Autodesk Fusion 360 part; units mm, degrees
note: some values were not read from the file. Set by a fixed rule: the direction of a hole.
(part 2 of 10)
  line L984 (55.9165, 3.84) -> (55.9165, 5.94)
  line L985 (53.6861, 6.8639) -> (53.4029, 6.44)
  line L986 (53.3035, 5.94) -> (53.3035, 5.94)
  line L987 (53.3035, 3.84) -> (53.3035, 3.84)
  line L988 (55.8171, 6.44) -> (55.5339, 6.8639)
  line L989 (55.5339, 6.8639) -> (55.11, 7.1471)
  line L990 (53.4029, 6.44) -> (53.3035, 5.94)
  line L991 (53.3035, 5.94) -> (53.3035, 3.84)
  line L992 (53.4029, 3.34) -> (53.6861, 2.9161)
  line L993 (55.11, 2.6329) -> (55.5339, 2.9161)
  line L994 (55.9165, 5.94) -> (55.9165, 5.94)
  line L995 (54.61, 7.2465) -> (54.11, 7.1471)
  line L996 (55.11, 7.1471) -> (54.61, 7.2465)
  line L997 (55.5339, 2.9161) -> (55.8171, 3.34)
  line L998 (53.3035, 3.84) -> (53.4029, 3.34)
  line L999 (96.49, 12.1015) -> (96.49, 12.1015)
  line L1000 (94.39, 9.4885) -> (96.49, 9.4885)
  line L1001 (93.1829, 11.295) -> (93.0835, 10.795)
  line L1002 (93.4661, 11.7189) -> (93.1829, 11.295)
  line L1003 (94.39, 12.1015) -> (93.89, 12.0021)
  line L1004 (93.89, 9.5879) -> (94.39, 9.4885)
  line L1005 (93.4661, 9.8711) -> (93.89, 9.5879)
  line L1006 (93.0835, 10.795) -> (93.1829, 10.295)
  line L1007 (93.1829, 10.295) -> (93.4661, 9.8711)
  line L1008 (96.99, 9.5879) -> (97.4139, 9.8711)
  line L1009 (97.6971, 10.295) -> (97.7965, 10.795)
  line L1010 (96.99, 12.0021) -> (96.49, 12.1015)
  line L1011 (96.49, 12.1015) -> (94.39, 12.1015)
  line L1012 (96.49, 9.4885) -> (96.49, 9.4885)
  line L1013 (94.39, 12.1015) -> (94.39, 12.1015)
  line L1014 (97.4139, 9.8711) -> (97.6971, 10.295)
  line L1015 (97.7965, 10.795) -> (97.6971, 11.295)
  line L1016 (93.89, 12.0021) -> (93.4661, 11.7189)
  line L1017 (94.39, 9.4885) -> (94.39, 9.4885)
  line L1018 (96.49, 9.4885) -> (96.99, 9.5879)
  line L1019 (97.4139, 11.7189) -> (96.99, 12.0021)
  line L1020 (97.6971, 11.295) -> (97.4139, 11.7189)
  line L1021 (67.81, 2.6329) -> (68.2339, 2.9161)
  line L1022 (67.31, 2.5335) -> (67.81, 2.6329)
  line L1023 (66.1029, 3.34) -> (66.3861, 2.9161)
  line L1024 (68.2339, 2.9161) -> (68.5171, 3.34)
  line L1025 (66.3861, 6.8639) -> (66.1029, 6.44)
  line L1026 (68.6165, 3.84) -> (68.6165, 3.84)
  line L1027 (66.3861, 2.9161) -> (66.81, 2.6329)
  line L1028 (67.31, 7.2465) -> (66.81, 7.1471)
  line L1029 (68.5171, 3.34) -> (68.6165, 3.84)
  line L1030 (66.0035, 5.94) -> (66.0035, 3.84)
  line L1031 (66.81, 2.6329) -> (67.31, 2.5335)
  line L1032 (68.6165, 5.94) -> (68.6165, 5.94)
  line L1033 (66.81, 7.1471) -> (66.3861, 6.8639)
  line L1034 (66.0035, 3.84) -> (66.0035, 3.84)
  line L1035 (67.81, 7.1471) -> (67.31, 7.2465)
  line L1036 (68.6165, 3.84) -> (68.6165, 5.94)
  line L1037 (66.1029, 6.44) -> (66.0035, 5.94)
  line L1038 (66.0035, 3.84) -> (66.1029, 3.34)
  line L1039 (66.0035, 5.94) -> (66.0035, 5.94)
  line L1040 (68.5171, 6.44) -> (68.2339, 6.8639)
  line L1041 (68.6165, 5.94) -> (68.5171, 6.44)
  line L1042 (68.2339, 6.8639) -> (67.81, 7.1471)
  line L1043 (41.9076, 68.8233) -> (41.9076, 68.8233)
  line L1044 (43.1725, 69.5114) -> (43.1997, 69.6484)
  line L1045 (43.1997, 70.1154) -> (43.1997, 70.1154)
  line L1046 (41.6544, 68.9282) -> (41.7706, 68.8506)
  line L1047 (43.1997, 69.6484) -> (43.1997, 70.1154)
  line L1048 (42.6278, 68.9282) -> (42.6278, 68.9282)
  line L1049 (41.7706, 68.8506) -> (41.9076, 68.8233)
  line L1050 (42.6278, 70.8356) -> (42.5117, 70.9132)
  line L1051 (43.0948, 70.3686) -> (43.0948, 70.3686)
  line L1052 (41.1874, 69.3952) -> (41.6544, 68.9282)
  line L1053 (41.1098, 70.2525) -> (41.0825, 70.1154)
  line L1054 (41.9076, 68.8233) -> (42.3746, 68.8233)
  line L1055 (43.1725, 70.2525) -> (43.0948, 70.3686)
  line L1056 (43.1997, 69.6484) -> (43.1997, 69.6484)
  line L1057 (42.3746, 68.8233) -> (42.5117, 68.8506)
  line L1058 (42.3746, 68.8233) -> (42.3746, 68.8233)
  line L1059 (43.1997, 70.1154) -> (43.1725, 70.2525)
  line L1060 (41.6544, 68.9282) -> (41.6544, 68.9282)
  line L1061 (41.0825, 69.6484) -> (41.1098, 69.5114)
  line L1062 (42.5117, 70.9132) -> (42.3746, 70.9405)
  line L1063 (43.0948, 70.3686) -> (42.6278, 70.8356)
  line L1064 (41.0825, 70.1154) -> (41.0825, 69.6484)
  line L1065 (41.6544, 70.8356) -> (41.1874, 70.3686)
  line L1066 (41.1874, 69.3952) -> (41.1874, 69.3952)
  line L1067 (41.6544, 70.8356) -> (41.6544, 70.8356)
  line L1068 (41.7706, 70.9132) -> (41.6544, 70.8356)
  line L1069 (42.3746, 70.9405) -> (42.3746, 70.9405)
  line L1070 (41.0825, 70.1154) -> (41.0825, 70.1154)
  line L1071 (41.1874, 70.3686) -> (41.1874, 70.3686)
  line L1072 (42.5117, 68.8506) -> (42.6278, 68.9282)
  line L1073 (41.1098, 69.5114) -> (41.1874, 69.3952)
  line L1074 (41.1874, 70.3686) -> (41.1098, 70.2525)
  line L1075 (41.0825, 69.6484) -> (41.0825, 69.6484)
  line L1076 (42.3746, 70.9405) -> (41.9076, 70.9405)
  line L1077 (41.9076, 70.9405) -> (41.9076, 70.9405)
  line L1078 (42.6278, 70.8356) -> (42.6278, 70.8356)
  line L1079 (43.0948, 69.3952) -> (43.1725, 69.5114)
  line L1080 (42.6278, 68.9282) -> (43.0948, 69.3952)
  line L1081 (41.9076, 70.9405) -> (41.7706, 70.9132)
  line L1082 (43.0948, 69.3952) -> (43.0948, 69.3952)
  line L1083 (35.9106, 76.5794) -> (35.9882, 76.6956)
  line L1084 (33.9256, 76.6956) -> (34.0032, 76.5794)
  line L1085 (35.4436, 78.0198) -> (35.4436, 78.0198)
  line L1086 (35.3275, 76.0348) -> (35.4436, 76.1124)
  line L1087 (34.4702, 76.1124) -> (34.4702, 76.1124)
  line L1088 (34.4702, 76.1124) -> (34.5864, 76.0348)
  line L1089 (35.1904, 78.1247) -> (35.1904, 78.1247)
  line L1090 (34.0032, 76.5794) -> (34.4702, 76.1124)
  line L1091 (35.9882, 76.6956) -> (36.0155, 76.8326)
  line L1092 (35.4436, 78.0198) -> (35.3275, 78.0975)
  line L1093 (35.4436, 76.1124) -> (35.9106, 76.5794)
  line L1094 (33.9256, 77.4367) -> (33.8983, 77.2996)
  line L1095 (34.7234, 76.0075) -> (34.7234, 76.0075)
  line L1096 (35.9106, 76.5794) -> (35.9106, 76.5794)
  line L1097 (35.9106, 77.5528) -> (35.9106, 77.5528)
  line L1098 (36.0155, 76.8326) -> (36.0155, 76.8326)
  line L1099 (34.0032, 77.5528) -> (33.9256, 77.4367)
  line L1100 (34.4702, 78.0198) -> (34.4702, 78.0198)
  line L1101 (36.0155, 77.2996) -> (35.9882, 77.4367)
  line L1102 (34.7234, 78.1247) -> (34.7234, 78.1247)
  line L1103 (35.3275, 78.0975) -> (35.1904, 78.1247)
  line L1104 (33.8983, 76.8326) -> (33.8983, 76.8326)
  line L1105 (35.1904, 78.1247) -> (34.7234, 78.1247)
  line L1106 (34.7234, 76.0075) -> (35.1904, 76.0075)
  line L1107 (35.9882, 77.4367) -> (35.9106, 77.5528)
  line L1108 (34.4702, 78.0198) -> (34.0032, 77.5528)
  line L1109 (36.0155, 77.2996) -> (36.0155, 77.2996)
  line L1110 (33.8983, 77.2996) -> (33.8983, 77.2996)
  line L1111 (33.8983, 77.2996) -> (33.8983, 76.8326)
  line L1112 (35.9106, 77.5528) -> (35.4436, 78.0198)
  line L1113 (35.1904, 76.0075) -> (35.1904, 76.0075)
  line L1114 (35.1904, 76.0075) -> (35.3275, 76.0348)
  line L1115 (33.8983, 76.8326) -> (33.9256, 76.6956)
  line L1116 (36.0155, 76.8326) -> (36.0155, 77.2996)
  line L1117 (34.7234, 78.1247) -> (34.5864, 78.0975)
  line L1118 (34.5864, 76.0348) -> (34.7234, 76.0075)
  line L1119 (34.0032, 76.5794) -> (34.0032, 76.5794)
  line L1120 (34.0032, 77.5528) -> (34.0032, 77.5528)
  line L1121 (34.5864, 78.0975) -> (34.4702, 78.0198)
  line L1122 (92.0234, 77.1136) -> (91.9073, 77.1913)
  line L1123 (90.4215, 76.5302) -> (90.4215, 75.8698)
  line L1124 (90.8566, 75.2864) -> (90.8566, 75.2864)
  line L1125 (90.9727, 77.1913) -> (90.8566, 77.1136)
  line L1126 (90.8566, 75.2864) -> (90.9727, 75.2087)
  line L1127 (90.8566, 77.1136) -> (90.8566, 77.1136)
  line L1128 (90.9727, 75.2087) -> (91.1098, 75.1815)
  line L1129 (90.5264, 75.6166) -> (90.5264, 75.6166)
  line L1130 (91.7702, 77.2185) -> (91.7702, 77.2185)
  line L1131 (92.3536, 75.6166) -> (92.3536, 75.6166)
  line L1132 (90.4487, 76.6673) -> (90.4215, 76.5302)
  line L1133 (91.1098, 75.1815) -> (91.1098, 75.1815)
  line L1134 (91.7702, 75.1815) -> (91.9073, 75.2087)
  line L1135 (90.4215, 75.8698) -> (90.4215, 75.8698)
  line L1136 (91.1098, 77.2185) -> (90.9727, 77.1913)
  line L1137 (90.4487, 75.7327) -> (90.5264, 75.6166)
  line L1138 (90.5264, 76.7834) -> (90.5264, 76.7834)
  line L1139 (91.1098, 75.1815) -> (91.7702, 75.1815)
  line L1140 (92.4585, 75.8698) -> (92.4585, 76.5302)
  line L1141 (91.7702, 75.1815) -> (91.7702, 75.1815)
  line L1142 (90.5264, 75.6166) -> (90.8566, 75.2864)
  line L1143 (92.4313, 75.7327) -> (92.4585, 75.8698)
  line L1144 (90.4215, 76.5302) -> (90.4215, 76.5302)
  line L1145 (92.0234, 75.2864) -> (92.0234, 75.2864)
  line L1146 (92.3536, 75.6166) -> (92.4313, 75.7327)
  line L1147 (91.9073, 75.2087) -> (92.0234, 75.2864)
  line L1148 (92.0234, 75.2864) -> (92.3536, 75.6166)
  line L1149 (90.8566, 77.1136) -> (90.5264, 76.7834)
  line L1150 (92.4585, 76.5302) -> (92.4313, 76.6673)
  line L1151 (91.7702, 77.2185) -> (91.1098, 77.2185)
  line L1152 (92.3536, 76.7834) -> (92.0234, 77.1136)
  line L1153 (91.9073, 77.1913) -> (91.7702, 77.2185)
  line L1154 (90.5264, 76.7834) -> (90.4487, 76.6673)
  line L1155 (91.1098, 77.2185) -> (91.1098, 77.2185)
  line L1156 (92.4585, 75.8698) -> (92.4585, 75.8698)
  line L1157 (90.4215, 75.8698) -> (90.4487, 75.7327)
  line L1158 (92.4313, 76.6673) -> (92.3536, 76.7834)
  line L1159 (92.4585, 76.5302) -> (92.4585, 76.5302)
  line L1160 (92.3536, 76.7834) -> (92.3536, 76.7834)
  line L1161 (92.0234, 77.1136) -> (92.0234, 77.1136)
  line L1162 (77.7215, 75.8698) -> (77.7215, 75.8698)
  line L1163 (78.1566, 75.2864) -> (78.2727, 75.2087)
  line L1164 (77.7487, 75.7327) -> (77.8264, 75.6166)
  line L1165 (78.1566, 77.1136) -> (77.8264, 76.7834)
  line L1166 (77.8264, 75.6166) -> (78.1566, 75.2864)
  line L1167 (79.3234, 75.2864) -> (79.6536, 75.6166)
  line L1168 (77.8264, 76.7834) -> (77.7487, 76.6673)
  line L1169 (77.7215, 76.5302) -> (77.7215, 75.8698)
  line L1170 (79.0702, 77.2185) -> (78.4098, 77.2185)
  line L1171 (79.6536, 75.6166) -> (79.6536, 75.6166)
  line L1172 (78.1566, 77.1136) -> (78.1566, 77.1136)
  line L1173 (79.3234, 77.1136) -> (79.3234, 77.1136)
  line L1174 (78.1566, 75.2864) -> (78.1566, 75.2864)
  line L1175 (79.7313, 75.7327) -> (79.7585, 75.8698)
  line L1176 (78.4098, 75.1815) -> (78.4098, 75.1815)
  line L1177 (78.2727, 77.1913) -> (78.1566, 77.1136)
  line L1178 (77.8264, 75.6166) -> (77.8264, 75.6166)
  line L1179 (79.6536, 76.7834) -> (79.6536, 76.7834)
  line L1180 (79.6536, 75.6166) -> (79.7313, 75.7327)
  line L1181 (78.4098, 75.1815) -> (79.0702, 75.1815)
  line L1182 (78.2727, 75.2087) -> (78.4098, 75.1815)
  line L1183 (79.7585, 76.5302) -> (79.7313, 76.6673)
  line L1184 (79.7585, 76.5302) -> (79.7585, 76.5302)
  line L1185 (79.0702, 77.2185) -> (79.0702, 77.2185)
  line L1186 (79.3234, 77.1136) -> (79.2073, 77.1913)
  line L1187 (77.7215, 76.5302) -> (77.7215, 76.5302)
  line L1188 (79.7585, 75.8698) -> (79.7585, 75.8698)
  line L1189 (77.8264, 76.7834) -> (77.8264, 76.7834)
  line L1190 (79.3234, 75.2864) -> (79.3234, 75.2864)
  line L1191 (79.0702, 75.1815) -> (79.0702, 75.1815)
  line L1192 (77.7215, 75.8698) -> (77.7487, 75.7327)
  line L1193 (79.7585, 75.8698) -> (79.7585, 76.5302)
  line L1194 (77.7487, 76.6673) -> (77.7215, 76.5302)
  line L1195 (79.2073, 77.1913) -> (79.0702, 77.2185)
  line L1196 (78.4098, 77.2185) -> (78.2727, 77.1913)
  line L1197 (78.4098, 77.2185) -> (78.4098, 77.2185)
  line L1198 (79.7313, 76.6673) -> (79.6536, 76.7834)
  line L1199 (79.2073, 75.2087) -> (79.3234, 75.2864)
  line L1200 (79.0702, 75.1815) -> (79.2073, 75.2087)
  line L1201 (79.6536, 76.7834) -> (79.3234, 77.1136)
  line L1202 (81.8634, 75.2864) -> (81.8634, 75.2864)
  line L1203 (80.2887, 76.6673) -> (80.2615, 76.5302)
  line L1204 (82.1936, 75.6166) -> (82.1936, 75.6166)
  line L1205 (81.7473, 75.2087) -> (81.8634, 75.2864)
  line L1206 (82.2713, 76.6673) -> (82.1936, 76.7834)
  line L1207 (81.6102, 75.1815) -> (81.7473, 75.2087)
  line L1208 (80.9498, 77.2185) -> (80.9498, 77.2185)
  line L1209 (80.2615, 76.5302) -> (80.2615, 76.5302)
  line L1210 (80.8127, 75.2087) -> (80.9498, 75.1815)
  line L1211 (80.6966, 75.2864) -> (80.8127, 75.2087)
  line L1212 (80.9498, 75.1815) -> (80.9498, 75.1815)
  line L1213 (81.6102, 77.2185) -> (81.6102, 77.2185)
  line L1214 (80.6966, 75.2864) -> (80.6966, 75.2864)
  line L1215 (81.6102, 77.2185) -> (80.9498, 77.2185)
  line L1216 (81.8634, 75.2864) -> (82.1936, 75.6166)
  line L1217 (82.2985, 75.8698) -> (82.2985, 76.5302)
  line L1218 (80.2615, 76.5302) -> (80.2615, 75.8698)
  line L1219 (80.8127, 77.1913) -> (80.6966, 77.1136)
  line L1220 (81.8634, 77.1136) -> (81.8634, 77.1136)
  line L1221 (82.2985, 76.5302) -> (82.2713, 76.6673)
  line L1222 (81.8634, 77.1136) -> (81.7473, 77.1913)
  line L1223 (80.3664, 75.6166) -> (80.6966, 75.2864)
  line L1224 (81.6102, 75.1815) -> (81.6102, 75.1815)
  line L1225 (80.3664, 76.7834) -> (80.2887, 76.6673)
  line L1226 (80.9498, 75.1815) -> (81.6102, 75.1815)
  line L1227 (80.3664, 75.6166) -> (80.3664, 75.6166)
  line L1228 (80.6966, 77.1136) -> (80.6966, 77.1136)
  line L1229 (82.2985, 76.5302) -> (82.2985, 76.5302)
  line L1230 (80.2887, 75.7327) -> (80.3664, 75.6166)
  line L1231 (80.2615, 75.8698) -> (80.2887, 75.7327)
  line L1232 (80.9498, 77.2185) -> (80.8127, 77.1913)
  line L1233 (81.7473, 77.1913) -> (81.6102, 77.2185)
  line L1234 (82.1936, 76.7834) -> (81.8634, 77.1136)
  line L1235 (80.6966, 77.1136) -> (80.3664, 76.7834)
  line L1236 (80.2615, 75.8698) -> (80.2615, 75.8698)
  line L1237 (82.1936, 76.7834) -> (82.1936, 76.7834)
  line L1238 (82.2985, 75.8698) -> (82.2985, 75.8698)
  line L1239 (82.1936, 75.6166) -> (82.2713, 75.7327)
  line L1240 (80.3664, 76.7834) -> (80.3664, 76.7834)
  line L1241 (82.2713, 75.7327) -> (82.2985, 75.8698)
  line L1242 (89.7027, 15.5187) -> (89.8398, 15.4915)
  line L1243 (89.1515, 16.8402) -> (89.1515, 16.1798)
  line L1244 (89.5866, 17.4236) -> (89.2564, 17.0934)
  line L1245 (89.5866, 17.4236) -> (89.5866, 17.4236)
  line L1246 (89.7027, 17.5013) -> (89.5866, 17.4236)
  line L1247 (90.6373, 17.5013) -> (90.5002, 17.5285)
  line L1248 (89.2564, 15.9266) -> (89.2564, 15.9266)
  line L1249 (89.1787, 16.9773) -> (89.1515, 16.8402)
  line L1250 (89.8398, 17.5285) -> (89.7027, 17.5013)
  line L1251 (89.2564, 17.0934) -> (89.1787, 16.9773)
  line L1252 (89.2564, 17.0934) -> (89.2564, 17.0934)
  line L1253 (89.1515, 16.1798) -> (89.1787, 16.0427)
  line L1254 (89.1515, 16.1798) -> (89.1515, 16.1798)
  line L1255 (91.1885, 16.8402) -> (91.1613, 16.9773)
  line L1256 (91.0836, 17.0934) -> (90.7534, 17.4236)
  line L1257 (91.1885, 16.1798) -> (91.1885, 16.1798)
  line L1258 (90.7534, 15.5964) -> (91.0836, 15.9266)
  line L1259 (90.7534, 17.4236) -> (90.6373, 17.5013)
  line L1260 (91.1613, 16.9773) -> (91.0836, 17.0934)
  line L1261 (89.8398, 15.4915) -> (90.5002, 15.4915)
  line L1262 (90.5002, 15.4915) -> (90.6373, 15.5187)
  line L1263 (89.5866, 15.5964) -> (89.5866, 15.5964)
  line L1264 (91.1885, 16.8402) -> (91.1885, 16.8402)
  line L1265 (89.8398, 15.4915) -> (89.8398, 15.4915)
  line L1266 (91.0836, 17.0934) -> (91.0836, 17.0934)
  line L1267 (90.7534, 15.5964) -> (90.7534, 15.5964)
  line L1268 (90.5002, 17.5285) -> (90.5002, 17.5285)
  line L1269 (90.5002, 15.4915) -> (90.5002, 15.4915)
  line L1270 (89.2564, 15.9266) -> (89.5866, 15.5964)
  line L1271 (90.6373, 15.5187) -> (90.7534, 15.5964)
  line L1272 (89.1787, 16.0427) -> (89.2564, 15.9266)
  line L1273 (91.1613, 16.0427) -> (91.1885, 16.1798)
  line L1274 (89.1515, 16.8402) -> (89.1515, 16.8402)
  line L1275 (89.5866, 15.5964) -> (89.7027, 15.5187)
  line L1276 (89.8398, 17.5285) -> (89.8398, 17.5285)
  line L1277 (91.0836, 15.9266) -> (91.0836, 15.9266)
  line L1278 (91.1885, 16.1798) -> (91.1885, 16.8402)
  line L1279 (91.0836, 15.9266) -> (91.1613, 16.0427)
  line L1280 (90.7534, 17.4236) -> (90.7534, 17.4236)
  line L1281 (90.5002, 17.5285) -> (89.8398, 17.5285)
  line L1282 (66.9798, 15.4915) -> (66.9798, 15.4915)
  line L1283 (66.2915, 16.1798) -> (66.3187, 16.0427)
  line L1284 (68.3285, 16.1798) -> (68.3285, 16.1798)
  line L1285 (68.2236, 17.0934) -> (67.8934, 17.4236)
  line L1286 (66.8427, 17.5013) -> (66.7266, 17.4236)
  line L1287 (66.3964, 17.0934) -> (66.3964, 17.0934)
  line L1288 (68.2236, 17.0934) -> (68.2236, 17.0934)
  line L1289 (68.2236, 15.9266) -> (68.2236, 15.9266)
  line L1290 (67.6402, 17.5285) -> (66.9798, 17.5285)
  line L1291 (68.3285, 16.1798) -> (68.3285, 16.8402)
  line L1292 (66.9798, 17.5285) -> (66.9798, 17.5285)
  line L1293 (67.6402, 15.4915) -> (67.7773, 15.5187)
  line L1294 (67.6402, 17.5285) -> (67.6402, 17.5285)
  line L1295 (67.7773, 15.5187) -> (67.8934, 15.5964)
  line L1296 (67.8934, 17.4236) -> (67.8934, 17.4236)
  line L1297 (68.2236, 15.9266) -> (68.3013, 16.0427)
  line L1298 (66.2915, 16.1798) -> (66.2915, 16.1798)
  line L1299 (66.2915, 16.8402) -> (66.2915, 16.8402)
  line L1300 (67.6402, 15.4915) -> (67.6402, 15.4915)
  line L1301 (66.3964, 17.0934) -> (66.3187, 16.9773)
  line L1302 (68.3013, 16.0427) -> (68.3285, 16.1798)
  line L1303 (66.7266, 15.5964) -> (66.8427, 15.5187)
  line L1304 (66.9798, 15.4915) -> (67.6402, 15.4915)
  line L1305 (67.7773, 17.5013) -> (67.6402, 17.5285)
  line L1306 (66.9798, 17.5285) -> (66.8427, 17.5013)
  line L1307 (66.8427, 15.5187) -> (66.9798, 15.4915)
  line L1308 (67.8934, 17.4236) -> (67.7773, 17.5013)
  line L1309 (66.2915, 16.8402) -> (66.2915, 16.1798)
  line L1310 (67.8934, 15.5964) -> (68.2236, 15.9266)
  line L1311 (66.3187, 16.9773) -> (66.2915, 16.8402)
  line L1312 (68.3013, 16.9773) -> (68.2236, 17.0934)
  line L1313 (66.3964, 15.9266) -> (66.3964, 15.9266)
  line L1314 (66.7266, 17.4236) -> (66.3964, 17.0934)
  line L1315 (68.3285, 16.8402) -> (68.3013, 16.9773)
  line L1316 (68.3285, 16.8402) -> (68.3285, 16.8402)
  line L1317 (67.8934, 15.5964) -> (67.8934, 15.5964)
  line L1318 (66.3187, 16.0427) -> (66.3964, 15.9266)
  line L1319 (66.7266, 17.4236) -> (66.7266, 17.4236)
  line L1320 (66.7266, 15.5964) -> (66.7266, 15.5964)
  line L1321 (66.3964, 15.9266) -> (66.7266, 15.5964)
  line L1322 (78.4098, 15.4915) -> (79.0702, 15.4915)
  line L1323 (79.6536, 17.0934) -> (79.6536, 17.0934)
  line L1324 (78.2727, 17.5013) -> (78.1566, 17.4236)
  line L1325 (79.6536, 15.9266) -> (79.6536, 15.9266)
  line L1326 (79.3234, 17.4236) -> (79.3234, 17.4236)
  line L1327 (78.4098, 17.5285) -> (78.4098, 17.5285)
  line L1328 (79.6536, 17.0934) -> (79.3234, 17.4236)
  line L1329 (79.7313, 16.9773) -> (79.6536, 17.0934)
  line L1330 (77.7215, 16.1798) -> (77.7215, 16.1798)
  line L1331 (79.0702, 17.5285) -> (79.0702, 17.5285)
  line L1332 (79.7585, 16.8402) -> (79.7585, 16.8402)
  line L1333 (77.7487, 16.0427) -> (77.8264, 15.9266)
  line L1334 (77.7215, 16.8402) -> (77.7215, 16.8402)
  line L1335 (79.0702, 15.4915) -> (79.2073, 15.5187)
  line L1336 (79.3234, 17.4236) -> (79.2073, 17.5013)
  line L1337 (77.7487, 16.9773) -> (77.7215, 16.8402)
  line L1338 (79.3234, 15.5964) -> (79.3234, 15.5964)
  line L1339 (77.7215, 16.8402) -> (77.7215, 16.1798)
  line L1340 (79.7585, 16.1798) -> (79.7585, 16.8402)
  line L1341 (79.2073, 15.5187) -> (79.3234, 15.5964)
  line L1342 (78.1566, 15.5964) -> (78.2727, 15.5187)
  line L1343 (79.7313, 16.0427) -> (79.7585, 16.1798)
  line L1344 (79.7585, 16.1798) -> (79.7585, 16.1798)
  line L1345 (78.1566, 17.4236) -> (78.1566, 17.4236)
  line L1346 (79.3234, 15.5964) -> (79.6536, 15.9266)
  line L1347 (78.1566, 17.4236) -> (77.8264, 17.0934)
  line L1348 (78.4098, 15.4915) -> (78.4098, 15.4915)
  line L1349 (78.1566, 15.5964) -> (78.1566, 15.5964)
  line L1350 (79.6536, 15.9266) -> (79.7313, 16.0427)
  line L1351 (77.7215, 16.1798) -> (77.7487, 16.0427)
  line L1352 (78.2727, 15.5187) -> (78.4098, 15.4915)
  line L1353 (77.8264, 15.9266) -> (78.1566, 15.5964)
  line L1354 (78.4098, 17.5285) -> (78.2727, 17.5013)
  line L1355 (79.0702, 15.4915) -> (79.0702, 15.4915)
  line L1356 (79.7585, 16.8402) -> (79.7313, 16.9773)
  line L1357 (77.8264, 17.0934) -> (77.8264, 17.0934)
  line L1358 (77.8264, 17.0934) -> (77.7487, 16.9773)
  line L1359 (77.8264, 15.9266) -> (77.8264, 15.9266)
  line L1360 (79.0702, 17.5285) -> (78.4098, 17.5285)
  line L1361 (79.2073, 17.5013) -> (79.0702, 17.5285)
  line L1362 (89.5866, 21.2336) -> (89.2564, 20.9034)
  line L1363 (89.1515, 20.6502) -> (89.1515, 19.9898)
  line L1364 (89.5866, 21.2336) -> (89.5866, 21.2336)
  line L1365 (89.2564, 20.9034) -> (89.1787, 20.7873)
  line L1366 (90.5002, 19.3015) -> (90.5002, 19.3015)
  line L1367 (89.8398, 19.3015) -> (89.8398, 19.3015)
  line L1368 (89.1515, 19.9898) -> (89.1515, 19.9898)
  line L1369 (91.0836, 19.7366) -> (91.0836, 19.7366)
  line L1370 (89.2564, 19.7366) -> (89.5866, 19.4064)
  line L1371 (89.8398, 19.3015) -> (90.5002, 19.3015)
  line L1372 (89.2564, 20.9034) -> (89.2564, 20.9034)
  line L1373 (89.1787, 19.8527) -> (89.2564, 19.7366)
  line L1374 (89.1515, 19.9898) -> (89.1787, 19.8527)
  line L1375 (91.1885, 20.6502) -> (91.1885, 20.6502)
  line L1376 (89.1787, 20.7873) -> (89.1515, 20.6502)
  line L1377 (89.1515, 20.6502) -> (89.1515, 20.6502)
  line L1378 (89.5866, 19.4064) -> (89.7027, 19.3287)
  line L1379 (89.2564, 19.7366) -> (89.2564, 19.7366)
  line L1380 (89.5866, 19.4064) -> (89.5866, 19.4064)
  line L1381 (91.1613, 19.8527) -> (91.1885, 19.9898)
  line L1382 (89.7027, 19.3287) -> (89.8398, 19.3015)
  line L1383 (90.5002, 19.3015) -> (90.6373, 19.3287)
  line L1384 (90.7534, 21.2336) -> (90.7534, 21.2336)
  line L1385 (90.7534, 21.2336) -> (90.6373, 21.3113)
  line L1386 (90.6373, 19.3287) -> (90.7534, 19.4064)
  line L1387 (91.0836, 20.9034) -> (90.7534, 21.2336)
  line L1388 (89.7027, 21.3113) -> (89.5866, 21.2336)
  line L1389 (89.8398, 21.3385) -> (89.8398, 21.3385)
  line L1390 (90.7534, 19.4064) -> (90.7534, 19.4064)
  line L1391 (90.5002, 21.3385) -> (89.8398, 21.3385)
  line L1392 (90.6373, 21.3113) -> (90.5002, 21.3385)
  line L1393 (91.0836, 19.7366) -> (91.1613, 19.8527)
  line L1394 (91.1885, 20.6502) -> (91.1613, 20.7873)
  line L1395 (91.0836, 20.9034) -> (91.0836, 20.9034)
  line L1396 (90.5002, 21.3385) -> (90.5002, 21.3385)
  line L1397 (90.7534, 19.4064) -> (91.0836, 19.7366)
  line L1398 (91.1613, 20.7873) -> (91.0836, 20.9034)
  line L1399 (89.8398, 21.3385) -> (89.7027, 21.3113)
  line L1400 (91.1885, 19.9898) -> (91.1885, 19.9898)
  line L1401 (91.1885, 19.9898) -> (91.1885, 20.6502)
  line L1402 (34.5687, 30.9473) -> (34.5415, 30.8102)
  line L1403 (34.9766, 31.3936) -> (34.6464, 31.0634)
  line L1404 (36.1434, 31.3936) -> (36.0273, 31.4713)
  line L1405 (34.5415, 30.1498) -> (34.5415, 30.1498)
  line L1406 (36.5785, 30.1498) -> (36.5785, 30.8102)
  line L1407 (36.4736, 31.0634) -> (36.1434, 31.3936)
  line L1408 (35.8902, 31.4985) -> (35.2298, 31.4985)
  line L1409 (36.1434, 31.3936) -> (36.1434, 31.3936)
  line L1410 (36.5785, 30.1498) -> (36.5785, 30.1498)
  line L1411 (34.5415, 30.1498) -> (34.5687, 30.0127)
  line L1412 (34.6464, 31.0634) -> (34.5687, 30.9473)
  line L1413 (36.4736, 29.8966) -> (36.4736, 29.8966)
  line L1414 (34.6464, 29.8966) -> (34.9766, 29.5664)
  line L1415 (34.5687, 30.0127) -> (34.6464, 29.8966)
  line L1416 (36.1434, 29.5664) -> (36.1434, 29.5664)
  line L1417 (36.5513, 30.0127) -> (36.5785, 30.1498)
  line L1418 (36.1434, 29.5664) -> (36.4736, 29.8966)
  line L1419 (34.9766, 29.5664) -> (34.9766, 29.5664)
  line L1420 (36.5785, 30.8102) -> (36.5513, 30.9473)
  line L1421 (35.8902, 29.4615) -> (36.0273, 29.4887)
  line L1422 (35.8902, 31.4985) -> (35.8902, 31.4985)
  line L1423 (36.0273, 31.4713) -> (35.8902, 31.4985)
  line L1424 (35.2298, 31.4985) -> (35.2298, 31.4985)
  line L1425 (35.2298, 31.4985) -> (35.0927, 31.4713)
  line L1426 (35.0927, 29.4887) -> (35.2298, 29.4615)
  line L1427 (36.5513, 30.9473) -> (36.4736, 31.0634)
  line L1428 (35.8902, 29.4615) -> (35.8902, 29.4615)
  line L1429 (34.9766, 31.3936) -> (34.9766, 31.3936)
  line L1430 (34.9766, 29.5664) -> (35.0927, 29.4887)
  line L1431 (35.0927, 31.4713) -> (34.9766, 31.3936)
  line L1432 (35.2298, 29.4615) -> (35.2298, 29.4615)
  line L1433 (34.6464, 31.0634) -> (34.6464, 31.0634)
  line L1434 (36.4736, 29.8966) -> (36.5513, 30.0127)
  line L1435 (36.5785, 30.8102) -> (36.5785, 30.8102)
  line L1436 (35.2298, 29.4615) -> (35.8902, 29.4615)
  line L1437 (34.6464, 29.8966) -> (34.6464, 29.8966)
  line L1438 (34.5415, 30.8102) -> (34.5415, 30.8102)
  line L1439 (36.0273, 29.4887) -> (36.1434, 29.5664)
  line L1440 (34.5415, 30.8102) -> (34.5415, 30.1498)
  line L1441 (36.4736, 31.0634) -> (36.4736, 31.0634)
  line L1442 (91.1613, 30.0127) -> (91.1885, 30.1498)
  line L1443 (91.1885, 30.1498) -> (91.1885, 30.1498)
  line L1444 (89.1787, 30.9473) -> (89.1515, 30.8102)
  line L1445 (89.8398, 31.4985) -> (89.7027, 31.4713)
  line L1446 (89.5866, 31.3936) -> (89.5866, 31.3936)
  line L1447 (89.8398, 29.4615) -> (90.5002, 29.4615)
  line L1448 (89.2564, 31.0634) -> (89.1787, 30.9473)
  line L1449 (90.7534, 31.3936) -> (90.7534, 31.3936)
  line L1450 (91.1885, 30.1498) -> (91.1885, 30.8102)
  line L1451 (89.7027, 29.4887) -> (89.8398, 29.4615)
  line L1452 (91.0836, 31.0634) -> (90.7534, 31.3936)
  line L1453 (89.5866, 29.5664) -> (89.5866, 29.5664)
  line L1454 (89.8398, 31.4985) -> (89.8398, 31.4985)
  line L1455 (90.5002, 29.4615) -> (90.5002, 29.4615)
  line L1456 (89.2564, 29.8966) -> (89.2564, 29.8966)
  line L1457 (90.5002, 31.4985) -> (89.8398, 31.4985)
  line L1458 (91.0836, 31.0634) -> (91.0836, 31.0634)
  line L1459 (90.6373, 31.4713) -> (90.5002, 31.4985)
  line L1460 (91.1885, 30.8102) -> (91.1885, 30.8102)
  line L1461 (89.1787, 30.0127) -> (89.2564, 29.8966)
  line L1462 (89.5866, 31.3936) -> (89.2564, 31.0634)
  line L1463 (89.1515, 30.1498) -> (89.1515, 30.1498)
  line L1464 (89.2564, 29.8966) -> (89.5866, 29.5664)
  line L1465 (91.1613, 30.9473) -> (91.0836, 31.0634)
  line L1466 (89.5866, 29.5664) -> (89.7027, 29.4887)
  line L1467 (91.0836, 29.8966) -> (91.0836, 29.8966)
  line L1468 (90.6373, 29.4887) -> (90.7534, 29.5664)
  line L1469 (91.1885, 30.8102) -> (91.1613, 30.9473)
  line L1470 (91.0836, 29.8966) -> (91.1613, 30.0127)
  line L1471 (89.1515, 30.8102) -> (89.1515, 30.1498)
  line L1472 (89.2564, 31.0634) -> (89.2564, 31.0634)
  line L1473 (89.1515, 30.8102) -> (89.1515, 30.8102)
  line L1474 (90.5002, 29.4615) -> (90.6373, 29.4887)
  line L1475 (90.7534, 29.5664) -> (91.0836, 29.8966)
  line L1476 (89.7027, 31.4713) -> (89.5866, 31.3936)
  line L1477 (89.1515, 30.1498) -> (89.1787, 30.0127)
  line L1478 (89.8398, 29.4615) -> (89.8398, 29.4615)
  line L1479 (90.7534, 31.3936) -> (90.6373, 31.4713)
  line L1480 (90.5002, 31.4985) -> (90.5002, 31.4985)
  line L1481 (90.7534, 29.5664) -> (90.7534, 29.5664)
  line L1482 (67.8934, 21.2336) -> (67.7773, 21.3113)
  line L1483 (67.8934, 19.4064) -> (67.8934, 19.4064)
  line L1484 (68.2236, 20.9034) -> (67.8934, 21.2336)
  line L1485 (68.3285, 19.9898) -> (68.3285, 19.9898)
  line L1486 (68.2236, 19.7366) -> (68.2236, 19.7366)
  line L1487 (66.3964, 20.9034) -> (66.3964, 20.9034)
  line L1488 (67.6402, 21.3385) -> (66.9798, 21.3385)
  line L1489 (66.9798, 21.3385) -> (66.9798, 21.3385)
  line L1490 (66.2915, 20.6502) -> (66.2915, 19.9898)
  line L1491 (68.3285, 20.6502) -> (68.3285, 20.6502)
  line L1492 (66.8427, 21.3113) -> (66.7266, 21.2336)
  line L1493 (67.6402, 19.3015) -> (67.7773, 19.3287)
  line L1494 (66.7266, 21.2336) -> (66.7266, 21.2336)
  line L1495 (66.9798, 21.3385) -> (66.8427, 21.3113)
  line L1496 (68.3285, 20.6502) -> (68.3013, 20.7873)
  line L1497 (67.6402, 21.3385) -> (67.6402, 21.3385)
  line L1498 (67.8934, 21.2336) -> (67.8934, 21.2336)
  line L1499 (67.7773, 21.3113) -> (67.6402, 21.3385)
  line L1500 (66.2915, 20.6502) -> (66.2915, 20.6502)
  line L1501 (68.3285, 19.9898) -> (68.3285, 20.6502)
  line L1502 (67.8934, 19.4064) -> (68.2236, 19.7366)
  line L1503 (68.3013, 20.7873) -> (68.2236, 20.9034)
  line L1504 (67.6402, 19.3015) -> (67.6402, 19.3015)
  line L1505 (66.9798, 19.3015) -> (67.6402, 19.3015)
  line L1506 (66.3964, 19.7366) -> (66.7266, 19.4064)
  line L1507 (66.8427, 19.3287) -> (66.9798, 19.3015)
  line L1508 (66.7266, 19.4064) -> (66.8427, 19.3287)
  line L1509 (66.9798, 19.3015) -> (66.9798, 19.3015)
  line L1510 (68.3013, 19.8527) -> (68.3285, 19.9898)
  line L1511 (66.3964, 19.7366) -> (66.3964, 19.7366)
  line L1512 (66.7266, 19.4064) -> (66.7266, 19.4064)
  line L1513 (66.2915, 19.9898) -> (66.3187, 19.8527)
  line L1514 (66.3187, 19.8527) -> (66.3964, 19.7366)
  line L1515 (66.3187, 20.7873) -> (66.2915, 20.6502)
  line L1516 (66.2915, 19.9898) -> (66.2915, 19.9898)
  line L1517 (66.3964, 20.9034) -> (66.3187, 20.7873)
  line L1518 (68.2236, 19.7366) -> (68.3013, 19.8527)
  line L1519 (66.7266, 21.2336) -> (66.3964, 20.9034)
  line L1520 (67.7773, 19.3287) -> (67.8934, 19.4064)
  line L1521 (68.2236, 20.9034) -> (68.2236, 20.9034)
  line L1522 (77.8264, 31.0634) -> (77.7487, 30.9473)
  line L1523 (79.3234, 31.3936) -> (79.2073, 31.4713)
  line L1524 (79.7585, 30.1498) -> (79.7585, 30.1498)
  line L1525 (79.2073, 29.4887) -> (79.3234, 29.5664)
  line L1526 (77.7487, 30.9473) -> (77.7215, 30.8102)
  line L1527 (79.3234, 29.5664) -> (79.6536, 29.8966)
  line L1528 (79.6536, 29.8966) -> (79.6536, 29.8966)
  line L1529 (79.7585, 30.1498) -> (79.7585, 30.8102)
  line L1530 (77.8264, 29.8966) -> (77.8264, 29.8966)
  line L1531 (79.6536, 31.0634) -> (79.3234, 31.3936)
  line L1532 (77.8264, 31.0634) -> (77.8264, 31.0634)
  line L1533 (79.7585, 30.8102) -> (79.7313, 30.9473)
  line L1534 (78.4098, 31.4985) -> (78.2727, 31.4713)
  line L1535 (79.0702, 31.4985) -> (79.0702, 31.4985)
  line L1536 (77.8264, 29.8966) -> (78.1566, 29.5664)
  line L1537 (77.7215, 30.1498) -> (77.7215, 30.1498)
  line L1538 (77.7215, 30.1498) -> (77.7487, 30.0127)
  line L1539 (77.7487, 30.0127) -> (77.8264, 29.8966)
  line L1540 (78.1566, 29.5664) -> (78.1566, 29.5664)
  line L1541 (79.6536, 31.0634) -> (79.6536, 31.0634)
  line L1542 (78.2727, 29.4887) -> (78.4098, 29.4615)
  line L1543 (79.0702, 29.4615) -> (79.0702, 29.4615)
  line L1544 (79.0702, 29.4615) -> (79.2073, 29.4887)
  line L1545 (77.7215, 30.8102) -> (77.7215, 30.8102)
  line L1546 (78.1566, 29.5664) -> (78.2727, 29.4887)
  line L1547 (78.1566, 31.3936) -> (77.8264, 31.0634)
  line L1548 (79.3234, 29.5664) -> (79.3234, 29.5664)
  line L1549 (77.7215, 30.8102) -> (77.7215, 30.1498)
  line L1550 (78.2727, 31.4713) -> (78.1566, 31.3936)
  line L1551 (78.4098, 31.4985) -> (78.4098, 31.4985)
  line L1552 (78.1566, 31.3936) -> (78.1566, 31.3936)
  line L1553 (78.4098, 29.4615) -> (78.4098, 29.4615)
  line L1554 (79.2073, 31.4713) -> (79.0702, 31.4985)
  line L1555 (79.7313, 30.0127) -> (79.7585, 30.1498)
  line L1556 (79.3234, 31.3936) -> (79.3234, 31.3936)
  line L1557 (79.6536, 29.8966) -> (79.7313, 30.0127)
  line L1558 (79.0702, 31.4985) -> (78.4098, 31.4985)
  line L1559 (78.4098, 29.4615) -> (79.0702, 29.4615)
  line L1560 (79.7313, 30.9473) -> (79.6536, 31.0634)
  line L1561 (79.7585, 30.8102) -> (79.7585, 30.8102)
  line L1562 (36.5513, 19.8527) -> (36.5785, 19.9898)
  line L1563 (34.9766, 19.4064) -> (35.0927, 19.3287)
  line L1564 (36.5785, 20.6502) -> (36.5513, 20.7873)
  line L1565 (36.4736, 19.7366) -> (36.4736, 19.7366)
  line L1566 (36.0273, 19.3287) -> (36.1434, 19.4064)
  line L1567 (36.1434, 19.4064) -> (36.1434, 19.4064)
  line L1568 (36.1434, 19.4064) -> (36.4736, 19.7366)
  line L1569 (35.8902, 19.3015) -> (36.0273, 19.3287)
  line L1570 (35.8902, 19.3015) -> (35.8902, 19.3015)
  line L1571 (35.2298, 19.3015) -> (35.8902, 19.3015)
  line L1572 (35.2298, 19.3015) -> (35.2298, 19.3015)
  line L1573 (35.0927, 19.3287) -> (35.2298, 19.3015)
  line L1574 (34.5415, 20.6502) -> (34.5415, 20.6502)
  line L1575 (34.6464, 19.7366) -> (34.6464, 19.7366)
  line L1576 (34.6464, 19.7366) -> (34.9766, 19.4064)
  line L1577 (36.5513, 20.7873) -> (36.4736, 20.9034)
  line L1578 (36.1434, 21.2336) -> (36.0273, 21.3113)
  line L1579 (35.8902, 21.3385) -> (35.8902, 21.3385)
  line L1580 (34.5415, 19.9898) -> (34.5415, 19.9898)
  line L1581 (34.6464, 20.9034) -> (34.6464, 20.9034)
  line L1582 (36.4736, 20.9034) -> (36.4736, 20.9034)
  line L1583 (34.5415, 19.9898) -> (34.5687, 19.8527)
  line L1584 (34.5415, 20.6502) -> (34.5415, 19.9898)
  line L1585 (36.0273, 21.3113) -> (35.8902, 21.3385)
  line L1586 (34.5687, 19.8527) -> (34.6464, 19.7366)
  line L1587 (36.4736, 20.9034) -> (36.1434, 21.2336)
  line L1588 (36.1434, 21.2336) -> (36.1434, 21.2336)
  line L1589 (36.5785, 20.6502) -> (36.5785, 20.6502)
  line L1590 (36.5785, 19.9898) -> (36.5785, 20.6502)
  line L1591 (35.2298, 21.3385) -> (35.2298, 21.3385)
  line L1592 (35.2298, 21.3385) -> (35.0927, 21.3113)
  line L1593 (34.9766, 21.2336) -> (34.6464, 20.9034)
  line L1594 (34.6464, 20.9034) -> (34.5687, 20.7873)
  line L1595 (35.8902, 21.3385) -> (35.2298, 21.3385)
  line L1596 (35.0927, 21.3113) -> (34.9766, 21.2336)
  line L1597 (36.5785, 19.9898) -> (36.5785, 19.9898)
  line L1598 (34.9766, 19.4064) -> (34.9766, 19.4064)
  line L1599 (36.4736, 19.7366) -> (36.5513, 19.8527)
  line L1600 (34.5687, 20.7873) -> (34.5415, 20.6502)
  line L1601 (34.9766, 21.2336) -> (34.9766, 21.2336)
  line L1602 (77.7215, 19.9898) -> (77.7487, 19.8527)
  line L1603 (79.6536, 19.7366) -> (79.7313, 19.8527)
  line L1604 (78.4098, 19.3015) -> (78.4098, 19.3015)
  line L1605 (79.7585, 19.9898) -> (79.7585, 20.6502)
  line L1606 (79.0702, 19.3015) -> (79.0702, 19.3015)
  line L1607 (77.8264, 20.9034) -> (77.8264, 20.9034)
  line L1608 (79.7585, 19.9898) -> (79.7585, 19.9898)
  line L1609 (78.4098, 19.3015) -> (79.0702, 19.3015)
  line L1610 (79.3234, 21.2336) -> (79.3234, 21.2336)
  line L1611 (78.1566, 21.2336) -> (77.8264, 20.9034)
  line L1612 (79.0702, 19.3015) -> (79.2073, 19.3287)
  line L1613 (79.2073, 21.3113) -> (79.0702, 21.3385)
  line L1614 (78.4098, 21.3385) -> (78.4098, 21.3385)
  line L1615 (79.7313, 19.8527) -> (79.7585, 19.9898)
  line L1616 (79.6536, 20.9034) -> (79.6536, 20.9034)
  line L1617 (79.6536, 20.9034) -> (79.3234, 21.2336)
  line L1618 (79.7313, 20.7873) -> (79.6536, 20.9034)
  line L1619 (79.7585, 20.6502) -> (79.7313, 20.7873)
  line L1620 (77.7487, 20.7873) -> (77.7215, 20.6502)
  line L1621 (79.3234, 21.2336) -> (79.2073, 21.3113)
  line L1622 (78.1566, 21.2336) -> (78.1566, 21.2336)
  line L1623 (78.2727, 21.3113) -> (78.1566, 21.2336)
  line L1624 (79.0702, 21.3385) -> (79.0702, 21.3385)
  line L1625 (79.7585, 20.6502) -> (79.7585, 20.6502)
  line L1626 (79.3234, 19.4064) -> (79.6536, 19.7366)
  line L1627 (78.1566, 19.4064) -> (78.1566, 19.4064)
  line L1628 (77.7215, 19.9898) -> (77.7215, 19.9898)
  line L1629 (78.4098, 21.3385) -> (78.2727, 21.3113)
  line L1630 (77.8264, 19.7366) -> (78.1566, 19.4064)
  line L1631 (77.7487, 19.8527) -> (77.8264, 19.7366)
  line L1632 (77.7215, 20.6502) -> (77.7215, 20.6502)
  line L1633 (79.0702, 21.3385) -> (78.4098, 21.3385)
  line L1634 (77.8264, 19.7366) -> (77.8264, 19.7366)
  line L1635 (77.8264, 20.9034) -> (77.7487, 20.7873)
  line L1636 (78.2727, 19.3287) -> (78.4098, 19.3015)
  line L1637 (77.7215, 20.6502) -> (77.7215, 19.9898)
  line L1638 (78.1566, 19.4064) -> (78.2727, 19.3287)
  line L1639 (79.6536, 19.7366) -> (79.6536, 19.7366)
  line L1640 (79.2073, 19.3287) -> (79.3234, 19.4064)
  line L1641 (79.3234, 19.4064) -> (79.3234, 19.4064)
  line L1642 (18.5827, 77.8263) -> (18.4666, 77.7486)
  line L1643 (18.1364, 77.4184) -> (18.1364, 77.4184)
  line L1644 (19.9636, 76.2516) -> (19.9636, 76.2516)
  line L1645 (18.7198, 77.8535) -> (18.5827, 77.8263)
  line L1646 (18.0315, 76.5048) -> (18.0315, 76.5048)
  line L1647 (20.0685, 77.1652) -> (20.0413, 77.3023)
  line L1648 (19.6334, 75.9214) -> (19.6334, 75.9214)
  line L1649 (18.0315, 77.1652) -> (18.0315, 76.5048)
  line L1650 (20.0685, 76.5048) -> (20.0685, 77.1652)
  line L1651 (19.9636, 76.2516) -> (20.0413, 76.3677)
  line L1652 (18.1364, 76.2516) -> (18.1364, 76.2516)
  line L1653 (19.9636, 77.4184) -> (19.9636, 77.4184)
  line L1654 (18.4666, 77.7486) -> (18.1364, 77.4184)
  line L1655 (18.4666, 75.9214) -> (18.4666, 75.9214)
  line L1656 (19.3802, 77.8535) -> (18.7198, 77.8535)
  line L1657 (20.0413, 77.3023) -> (19.9636, 77.4184)
  line L1658 (18.5827, 75.8437) -> (18.7198, 75.8165)
  line L1659 (18.0587, 77.3023) -> (18.0315, 77.1652)
  line L1660 (19.3802, 75.8165) -> (19.5173, 75.8437)
  line L1661 (19.5173, 75.8437) -> (19.6334, 75.9214)
  line L1662 (18.7198, 75.8165) -> (19.3802, 75.8165)
  line L1663 (19.6334, 77.7486) -> (19.6334, 77.7486)
  line L1664 (19.6334, 77.7486) -> (19.5173, 77.8263)
  line L1665 (18.1364, 76.2516) -> (18.4666, 75.9214)
  line L1666 (18.4666, 75.9214) -> (18.5827, 75.8437)
  line L1667 (19.3802, 77.8535) -> (19.3802, 77.8535)
  line L1668 (19.9636, 77.4184) -> (19.6334, 77.7486)
  line L1669 (19.6334, 75.9214) -> (19.9636, 76.2516)
  line L1670 (18.0315, 77.1652) -> (18.0315, 77.1652)
  line L1671 (18.7198, 75.8165) -> (18.7198, 75.8165)
  line L1672 (18.7198, 77.8535) -> (18.7198, 77.8535)
  line L1673 (18.1364, 77.4184) -> (18.0587, 77.3023)
  line L1674 (18.4666, 77.7486) -> (18.4666, 77.7486)
  line L1675 (20.0413, 76.3677) -> (20.0685, 76.5048)
  line L1676 (18.0587, 76.3677) -> (18.1364, 76.2516)
  line L1677 (18.0315, 76.5048) -> (18.0587, 76.3677)
  line L1678 (19.3802, 75.8165) -> (19.3802, 75.8165)
  line L1679 (20.0685, 76.5048) -> (20.0685, 76.5048)
  line L1680 (20.0685, 77.1652) -> (20.0685, 77.1652)
  line L1681 (19.5173, 77.8263) -> (19.3802, 77.8535)
  line L1682 (53.8073, 31.4713) -> (53.6702, 31.4985)
  line L1683 (52.7566, 29.5664) -> (52.7566, 29.5664)
  line L1684 (52.4264, 31.0634) -> (52.3487, 30.9473)
  line L1685 (52.3487, 30.0127) -> (52.4264, 29.8966)
  line L1686 (53.6702, 31.4985) -> (53.6702, 31.4985)
  line L1687 (52.3215, 30.1498) -> (52.3215, 30.1498)
  line L1688 (53.0098, 29.4615) -> (53.6702, 29.4615)
  line L1689 (52.7566, 29.5664) -> (52.8727, 29.4887)
  line L1690 (53.0098, 29.4615) -> (53.0098, 29.4615)
  line L1691 (53.6702, 29.4615) -> (53.6702, 29.4615)
  line L1692 (52.3215, 30.8102) -> (52.3215, 30.1498)
  line L1693 (52.4264, 31.0634) -> (52.4264, 31.0634)
  line L1694 (52.3215, 30.8102) -> (52.3215, 30.8102)
  line L1695 (54.3313, 30.9473) -> (54.2536, 31.0634)
  line L1696 (53.8073, 29.4887) -> (53.9234, 29.5664)
  line L1697 (54.2536, 31.0634) -> (54.2536, 31.0634)
  line L1698 (54.3313, 30.0127) -> (54.3585, 30.1498)
  line L1699 (54.3585, 30.8102) -> (54.3585, 30.8102)
  line L1700 (52.4264, 29.8966) -> (52.4264, 29.8966)
  line L1701 (52.8727, 31.4713) -> (52.7566, 31.3936)
  line L1702 (53.6702, 29.4615) -> (53.8073, 29.4887)
  line L1703 (54.2536, 29.8966) -> (54.3313, 30.0127)
  line L1704 (53.9234, 29.5664) -> (54.2536, 29.8966)
  line L1705 (53.0098, 31.4985) -> (52.8727, 31.4713)
  line L1706 (53.6702, 31.4985) -> (53.0098, 31.4985)
  line L1707 (53.9234, 31.3936) -> (53.9234, 31.3936)
  line L1708 (53.9234, 29.5664) -> (53.9234, 29.5664)
  line L1709 (52.4264, 29.8966) -> (52.7566, 29.5664)
  line L1710 (54.2536, 31.0634) -> (53.9234, 31.3936)
  line L1711 (52.7566, 31.3936) -> (52.7566, 31.3936)
  line L1712 (54.2536, 29.8966) -> (54.2536, 29.8966)
  line L1713 (54.3585, 30.8102) -> (54.3313, 30.9473)
  line L1714 (52.3487, 30.9473) -> (52.3215, 30.8102)
  line L1715 (54.3585, 30.1498) -> (54.3585, 30.1498)
  line L1716 (54.3585, 30.1498) -> (54.3585, 30.8102)
  line L1717 (53.9234, 31.3936) -> (53.8073, 31.4713)
  line L1718 (52.8727, 29.4887) -> (53.0098, 29.4615)
  line L1719 (52.7566, 31.3936) -> (52.4264, 31.0634)
  line L1720 (52.3215, 30.1498) -> (52.3487, 30.0127)
  line L1721 (53.0098, 31.4985) -> (53.0098, 31.4985)
  line L1722 (48.5902, 29.4615) -> (48.5902, 29.4615)
  line L1723 (48.8434, 31.3936) -> (48.7273, 31.4713)
  line L1724 (47.6766, 29.5664) -> (47.6766, 29.5664)
  line L1725 (48.7273, 31.4713) -> (48.5902, 31.4985)
  line L1726 (47.3464, 31.0634) -> (47.3464, 31.0634)
  line L1727 (47.2415, 30.1498) -> (47.2687, 30.0127)
  line L1728 (47.3464, 31.0634) -> (47.2687, 30.9473)
  line L1729 (47.2415, 30.1498) -> (47.2415, 30.1498)
  line L1730 (49.2785, 30.8102) -> (49.2513, 30.9473)
  line L1731 (47.3464, 29.8966) -> (47.3464, 29.8966)
  line L1732 (49.2785, 30.8102) -> (49.2785, 30.8102)
  line L1733 (47.9298, 29.4615) -> (47.9298, 29.4615)
  line L1734 (47.2415, 30.8102) -> (47.2415, 30.1498)
  line L1735 (49.2785, 30.1498) -> (49.2785, 30.8102)
  line L1736 (49.1736, 29.8966) -> (49.2513, 30.0127)
  line L1737 (47.6766, 29.5664) -> (47.7927, 29.4887)
  line L1738 (48.7273, 29.4887) -> (48.8434, 29.5664)
  line L1739 (48.5902, 29.4615) -> (48.7273, 29.4887)
  line L1740 (49.1736, 31.0634) -> (49.1736, 31.0634)
  line L1741 (47.9298, 29.4615) -> (48.5902, 29.4615)
  line L1742 (48.8434, 31.3936) -> (48.8434, 31.3936)
  line L1743 (49.2513, 30.0127) -> (49.2785, 30.1498)
  line L1744 (47.6766, 31.3936) -> (47.3464, 31.0634)
  line L1745 (47.6766, 31.3936) -> (47.6766, 31.3936)
  line L1746 (49.1736, 31.0634) -> (48.8434, 31.3936)
  line L1747 (48.8434, 29.5664) -> (49.1736, 29.8966)
  line L1748 (49.2785, 30.1498) -> (49.2785, 30.1498)
  line L1749 (47.3464, 29.8966) -> (47.6766, 29.5664)
  line L1750 (47.7927, 31.4713) -> (47.6766, 31.3936)
  line L1751 (49.2513, 30.9473) -> (49.1736, 31.0634)
  line L1752 (47.9298, 31.4985) -> (47.9298, 31.4985)
  line L1753 (47.9298, 31.4985) -> (47.7927, 31.4713)
  line L1754 (48.5902, 31.4985) -> (47.9298, 31.4985)
  line L1755 (47.2415, 30.8102) -> (47.2415, 30.8102)
  line L1756 (49.1736, 29.8966) -> (49.1736, 29.8966)
  line L1757 (47.2687, 30.0127) -> (47.3464, 29.8966)
  line L1758 (48.5902, 31.4985) -> (48.5902, 31.4985)
  line L1759 (47.2687, 30.9473) -> (47.2415, 30.8102)
  line L1760 (48.8434, 29.5664) -> (48.8434, 29.5664)
  line L1761 (47.7927, 29.4887) -> (47.9298, 29.4615)
  line L1762 (47.6766, 19.4064) -> (47.7927, 19.3287)
  line L1763 (48.7273, 21.3113) -> (48.5902, 21.3385)
  line L1764 (47.2415, 19.9898) -> (47.2415, 19.9898)
  line L1765 (47.3464, 19.7366) -> (47.6766, 19.4064)
  line L1766 (49.2785, 20.6502) -> (49.2513, 20.7873)
  line L1767 (47.2415, 19.9898) -> (47.2687, 19.8527)
  line L1768 (47.6766, 21.2336) -> (47.3464, 20.9034)
  line L1769 (49.2785, 19.9898) -> (49.2785, 19.9898)
  line L1770 (47.9298, 21.3385) -> (47.9298, 21.3385)
  line L1771 (47.9298, 19.3015) -> (47.9298, 19.3015)
  line L1772 (48.8434, 19.4064) -> (48.8434, 19.4064)
  line L1773 (47.9298, 19.3015) -> (48.5902, 19.3015)
  line L1774 (48.7273, 19.3287) -> (48.8434, 19.4064)
  line L1775 (48.5902, 19.3015) -> (48.7273, 19.3287)
  line L1776 (48.5902, 19.3015) -> (48.5902, 19.3015)
  line L1777 (48.8434, 19.4064) -> (49.1736, 19.7366)
  line L1778 (47.6766, 19.4064) -> (47.6766, 19.4064)
  line L1779 (49.2513, 19.8527) -> (49.2785, 19.9898)
  line L1780 (47.2415, 20.6502) -> (47.2415, 19.9898)
  line L1781 (47.9298, 21.3385) -> (47.7927, 21.3113)
  line L1782 (49.1736, 20.9034) -> (48.8434, 21.2336)
  line L1783 (48.5902, 21.3385) -> (48.5902, 21.3385)
  line L1784 (48.8434, 21.2336) -> (48.8434, 21.2336)
  line L1785 (47.7927, 21.3113) -> (47.6766, 21.2336)
  line L1786 (47.3464, 20.9034) -> (47.3464, 20.9034)
  line L1787 (49.1736, 20.9034) -> (49.1736, 20.9034)
  line L1788 (49.1736, 19.7366) -> (49.1736, 19.7366)
  line L1789 (47.3464, 19.7366) -> (47.3464, 19.7366)
  line L1790 (49.2785, 19.9898) -> (49.2785, 20.6502)
  line L1791 (47.7927, 19.3287) -> (47.9298, 19.3015)
  line L1792 (47.2687, 19.8527) -> (47.3464, 19.7366)
  line L1793 (47.2415, 20.6502) -> (47.2415, 20.6502)
  line L1794 (47.2687, 20.7873) -> (47.2415, 20.6502)
  line L1795 (47.3464, 20.9034) -> (47.2687, 20.7873)
  line L1796 (48.8434, 21.2336) -> (48.7273, 21.3113)
  line L1797 (49.2785, 20.6502) -> (49.2785, 20.6502)
  line L1798 (49.2513, 20.7873) -> (49.1736, 20.9034)
  line L1799 (48.5902, 21.3385) -> (47.9298, 21.3385)
  line L1800 (47.6766, 21.2336) -> (47.6766, 21.2336)
  line L1801 (49.1736, 19.7366) -> (49.2513, 19.8527)
  line L1802 (54.3585, 20.6502) -> (54.3313, 20.7873)
  line L1803 (52.3487, 20.7873) -> (52.3215, 20.6502)
  line L1804 (52.7566, 21.2336) -> (52.4264, 20.9034)
  line L1805 (52.7566, 21.2336) -> (52.7566, 21.2336)
  line L1806 (53.0098, 21.3385) -> (52.8727, 21.3113)
  line L1807 (53.6702, 21.3385) -> (53.6702, 21.3385)
  line L1808 (54.2536, 20.9034) -> (53.9234, 21.2336)
  line L1809 (53.6702, 21.3385) -> (53.0098, 21.3385)
  line L1810 (52.8727, 21.3113) -> (52.7566, 21.2336)
  line L1811 (53.9234, 19.4064) -> (53.9234, 19.4064)
  line L1812 (54.3585, 20.6502) -> (54.3585, 20.6502)
  line L1813 (54.2536, 19.7366) -> (54.3313, 19.8527)
  line L1814 (54.2536, 20.9034) -> (54.2536, 20.9034)
  line L1815 (54.2536, 19.7366) -> (54.2536, 19.7366)
  line L1816 (53.9234, 19.4064) -> (54.2536, 19.7366)
  line L1817 (54.3313, 20.7873) -> (54.2536, 20.9034)
  line L1818 (54.3313, 19.8527) -> (54.3585, 19.9898)
  line L1819 (54.3585, 19.9898) -> (54.3585, 19.9898)
  line L1820 (54.3585, 19.9898) -> (54.3585, 20.6502)
  line L1821 (53.6702, 19.3015) -> (53.8073, 19.3287)
  line L1822 (53.8073, 21.3113) -> (53.6702, 21.3385)
  line L1823 (53.9234, 21.2336) -> (53.8073, 21.3113)
  line L1824 (53.0098, 21.3385) -> (53.0098, 21.3385)
  line L1825 (53.9234, 21.2336) -> (53.9234, 21.2336)
  line L1826 (53.8073, 19.3287) -> (53.9234, 19.4064)
  line L1827 (52.3215, 20.6502) -> (52.3215, 19.9898)
  line L1828 (52.8727, 19.3287) -> (53.0098, 19.3015)
  line L1829 (53.0098, 19.3015) -> (53.6702, 19.3015)
  line L1830 (52.7566, 19.4064) -> (52.7566, 19.4064)
  line L1831 (52.3215, 20.6502) -> (52.3215, 20.6502)
  line L1832 (52.3215, 19.9898) -> (52.3487, 19.8527)
  line L1833 (52.4264, 20.9034) -> (52.3487, 20.7873)
  line L1834 (53.0098, 19.3015) -> (53.0098, 19.3015)
  line L1835 (52.3215, 19.9898) -> (52.3215, 19.9898)
  line L1836 (53.6702, 19.3015) -> (53.6702, 19.3015)
  line L1837 (52.4264, 20.9034) -> (52.4264, 20.9034)
  line L1838 (52.4264, 19.7366) -> (52.7566, 19.4064)
  line L1839 (52.3487, 19.8527) -> (52.4264, 19.7366)
  line L1840 (52.7566, 19.4064) -> (52.8727, 19.3287)
  line L1841 (52.4264, 19.7366) -> (52.4264, 19.7366)
  line L1842 (7.9764, 77.4184) -> (7.9764, 77.4184)
  line L1843 (9.2202, 77.8535) -> (9.2202, 77.8535)
  line L1844 (9.9085, 77.1652) -> (9.9085, 77.1652)
  line L1845 (9.2202, 77.8535) -> (8.5598, 77.8535)
  line L1846 (8.5598, 77.8535) -> (8.4227, 77.8263)
  line L1847 (8.3066, 77.7486) -> (8.3066, 77.7486)
  line L1848 (9.3573, 77.8263) -> (9.2202, 77.8535)
  line L1849 (7.8715, 76.5048) -> (7.8987, 76.3677)
  line L1850 (7.8715, 76.5048) -> (7.8715, 76.5048)
  line L1851 (9.4734, 77.7486) -> (9.4734, 77.7486)
  line L1852 (8.5598, 75.8165) -> (9.2202, 75.8165)
  line L1853 (9.8813, 77.3023) -> (9.8036, 77.4184)
  line L1854 (7.9764, 76.2516) -> (8.3066, 75.9214)
  line L1855 (9.4734, 77.7486) -> (9.3573, 77.8263)
  line L1856 (8.5598, 75.8165) -> (8.5598, 75.8165)
  line L1857 (9.8036, 77.4184) -> (9.4734, 77.7486)
  line L1858 (9.9085, 77.1652) -> (9.8813, 77.3023)
  line L1859 (8.3066, 77.7486) -> (7.9764, 77.4184)
  line L1860 (7.8715, 77.1652) -> (7.8715, 76.5048)
  line L1861 (8.4227, 75.8437) -> (8.5598, 75.8165)
  line L1862 (9.2202, 75.8165) -> (9.2202, 75.8165)
  line L1863 (9.8813, 76.3677) -> (9.9085, 76.5048)
  line L1864 (9.9085, 76.5048) -> (9.9085, 77.1652)
  line L1865 (9.9085, 76.5048) -> (9.9085, 76.5048)
  line L1866 (7.8987, 77.3023) -> (7.8715, 77.1652)
  line L1867 (9.3573, 75.8437) -> (9.4734, 75.9214)
  line L1868 (9.8036, 76.2516) -> (9.8813, 76.3677)
  line L1869 (7.8987, 76.3677) -> (7.9764, 76.2516)
  line L1870 (8.5598, 77.8535) -> (8.5598, 77.8535)
  line L1871 (9.2202, 75.8165) -> (9.3573, 75.8437)
  line L1872 (7.9764, 77.4184) -> (7.8987, 77.3023)
  line L1873 (7.8715, 77.1652) -> (7.8715, 77.1652)
  line L1874 (8.3066, 75.9214) -> (8.3066, 75.9214)
  line L1875 (9.4734, 75.9214) -> (9.4734, 75.9214)
  line L1876 (8.3066, 75.9214) -> (8.4227, 75.8437)
  line L1877 (7.9764, 76.2516) -> (7.9764, 76.2516)
  line L1878 (9.8036, 77.4184) -> (9.8036, 77.4184)
  line L1879 (9.4734, 75.9214) -> (9.8036, 76.2516)
  line L1880 (8.4227, 77.8263) -> (8.3066, 77.7486)
  line L1881 (9.8036, 76.2516) -> (9.8036, 76.2516)
  line L1882 (9.2464, 15.9266) -> (9.5766, 15.5964)
  line L1883 (9.8298, 15.4915) -> (9.8298, 15.4915)
  line L1884 (9.5766, 15.5964) -> (9.6927, 15.5187)
  line L1885 (11.1513, 16.9773) -> (11.0736, 17.0934)
  line L1886 (10.6273, 15.5187) -> (10.7434, 15.5964)
  line L1887 (10.7434, 15.5964) -> (11.0736, 15.9266)
  line L1888 (10.7434, 17.4236) -> (10.7434, 17.4236)
  line L1889 (11.0736, 17.0934) -> (11.0736, 17.0934)
  line L1890 (11.1785, 16.8402) -> (11.1785, 16.8402)
  line L1891 (11.1785, 16.8402) -> (11.1513, 16.9773)
  line L1892 (11.0736, 15.9266) -> (11.0736, 15.9266)
  line L1893 (10.7434, 15.5964) -> (10.7434, 15.5964)
  line L1894 (11.0736, 15.9266) -> (11.1513, 16.0427)
  line L1895 (11.1785, 16.1798) -> (11.1785, 16.8402)
  line L1896 (10.4902, 15.4915) -> (10.4902, 15.4915)
  line L1897 (9.6927, 15.5187) -> (9.8298, 15.4915)
  line L1898 (10.4902, 15.4915) -> (10.6273, 15.5187)
  line L1899 (9.8298, 15.4915) -> (10.4902, 15.4915)
  line L1900 (9.2464, 17.0934) -> (9.1687, 16.9773)
  line L1901 (9.5766, 17.4236) -> (9.2464, 17.0934)
  line L1902 (9.8298, 17.5285) -> (9.8298, 17.5285)
  line L1903 (11.0736, 17.0934) -> (10.7434, 17.4236)
  line L1904 (11.1513, 16.0427) -> (11.1785, 16.1798)
  line L1905 (10.4902, 17.5285) -> (10.4902, 17.5285)
  line L1906 (10.6273, 17.5013) -> (10.4902, 17.5285)
  line L1907 (9.1687, 16.9773) -> (9.1415, 16.8402)
  line L1908 (9.6927, 17.5013) -> (9.5766, 17.4236)
  line L1909 (9.5766, 15.5964) -> (9.5766, 15.5964)
  line L1910 (9.8298, 17.5285) -> (9.6927, 17.5013)
  line L1911 (10.4902, 17.5285) -> (9.8298, 17.5285)
  line L1912 (9.5766, 17.4236) -> (9.5766, 17.4236)